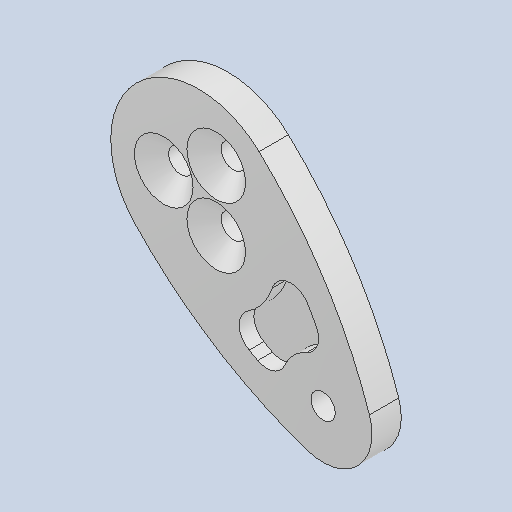
# Autodesk Inventor part: クランク_前
Saved by Autodesk Inventor 2023 (Build 270158030, 158C)
## iProperties
Created: 2022-01-08
Part Number: クランク_前
Material: Aluminum 2014-T6
Document SubType Name: Modeling
Designer: acps
Density: 2.78927 g/cm^3
Appearance: Satin
Author: acps
Autodesk Inventor part; units mm, degrees
ref_plane "YZ Plane" through (0, 0, 0) normal (1, 0, 0) x (0, 1, 0)
ref_plane "XZ Plane" through (0, 0, 0) normal (0, 1, 0) x (-1, 0, 0)
ref_plane "XY Plane" through (0, 0, 0) normal (0, 0, 1) x (1, 0, 0)
sketch "Sketch2" plane through (0, 0, 0) normal (0, 0, 1) x (1, 0, 0)
  line L0 (0, 0) -> (-12.7279, 12.7279) construction
  line L1 (0, 0) -> (18, 0) construction
  line L2 (0, 0) -> (-12.7279, 12.7279) construction
  line L3 (-3.5355, -3.5355) -> (-16.2635, 9.1924) construction
  line L4 (-9.1924, 16.2635) -> (3.5355, 3.5355) construction
  arc A0 (-3.5355, -3.5355) -> (-1.5844, -4.7423) centre (0, 0) ccw construction
  arc A1 (-9.1924, 16.2635) -> (-16.2635, 9.1924) centre (-12.7279, 12.7279) ccw
  arc A2 (-6.5476, 19.2704) -> (-19.2704, 6.5476) centre (-12.7279, 12.7279) ccw
  arc A3 (-19.2704, 6.5476) -> (-1.5844, -4.7423) centre (12.0821, 36.1644) ccw
  arc A4 (4.7423, 1.5844) -> (-6.5476, 19.2704) centre (-36.1644, -12.0821) ccw
  arc A5 (-3.9009, 10.972) -> (-6.5476, 19.2704) centre (-12.7279, 12.7279) ccw construction
  arc A6 (-6.364, 6.364) -> (-3.9009, 10.972) centre (-12.7279, 12.7279) ccw construction
  arc A7 (-10.972, 3.9009) -> (-6.364, 6.364) centre (-12.7279, 12.7279) ccw construction
  arc A8 (-19.2704, 6.5476) -> (-10.972, 3.9009) centre (-12.7279, 12.7279) ccw construction
  arc A9 (4.7423, 1.5844) -> (3.5355, 3.5355) centre (0, 0) ccw construction
  circle A10 centre (0, 0) radius 5
  circle A11 centre (0, 0) radius 3.025 construction
  circle A12 centre (0, 0) radius 1.25
  line L5 (0, 0) -> (-12.7279, 12.7279) construction
  line L6 (0, 0) -> (18, 0) construction
  line L7 (0, 0) -> (-12.7279, 12.7279) construction
  line L8 (-3.5355, -3.5355) -> (-16.2635, 9.1924) construction
  line L9 (-9.1924, 16.2635) -> (3.5355, 3.5355) construction
  arc A13 (-3.5355, -3.5355) -> (-1.5844, -4.7423) centre (0, 0) ccw construction
  arc A14 (-9.1924, 16.2635) -> (-16.2635, 9.1924) centre (-12.7279, 12.7279) ccw
  arc A15 (-6.5476, 19.2704) -> (-19.2704, 6.5476) centre (-12.7279, 12.7279) ccw
  circle A16 centre (-10.9381, 15.8279) radius 1.25
  circle A17 centre (-10.9381, 15.8279) radius 3.1 construction
  circle A18 centre (-16.3075, 12.7279) radius 1.25
  circle A19 centre (-16.3075, 12.7279) radius 3.1 construction
  circle A20 centre (-10.9381, 9.6279) radius 1.25
  circle A21 centre (-10.9381, 9.6279) radius 3.1 construction
  arc A22 (-19.2704, 6.5476) -> (-1.5844, -4.7423) centre (12.0821, 36.1644) ccw
  arc A23 (4.7423, 1.5844) -> (-6.5476, 19.2704) centre (-36.1644, -12.0821) ccw
  arc A24 (-3.9009, 10.972) -> (-6.5476, 19.2704) centre (-12.7279, 12.7279) ccw construction
  arc A25 (-6.364, 6.364) -> (-3.9009, 10.972) centre (-12.7279, 12.7279) ccw construction
  arc A26 (-10.972, 3.9009) -> (-6.364, 6.364) centre (-12.7279, 12.7279) ccw construction
  arc A27 (-19.2704, 6.5476) -> (-10.972, 3.9009) centre (-12.7279, 12.7279) ccw construction
  arc A28 (4.7423, 1.5844) -> (3.5355, 3.5355) centre (0, 0) ccw construction
  circle A29 centre (0, 0) radius 5
  circle A30 centre (0, 0) radius 3.025 construction
  circle A31 centre (0, 0) radius 1.25
  point P0 (-6.364, 6.364)
  point P1 (-11.1244, -0.1893)
  point P2 (-6.364, 6.364)
  point P3 (-11.1244, -0.1893)
  point P4 (4.7423, 1.5844)
  point P5 (-1.5844, -4.7423)
  dimension "d47" = 18
  dimension "d48" = 135
  dimension "d49" = 5
  dimension "d50" = 18
  dimension "d54" = 8
  dimension "d55" = 10
  dimension "d56" = 6.05
  dimension "d57" = 2.5
  dimension "d58" = 18
  dimension "d59" = 135
  dimension "d60" = 5
  dimension "d61" = 18
  dimension "d62" = 2.5
  dimension "d63" = 6.2
  dimension "d64" = 360
  dimension "d65" = 8
  dimension "d66" = 10
  dimension "d67" = 6.05
  dimension "d68" = 2.5
  constraints: 48 point on circle, 32 centre point, 24 end point, 17 tangent, 11 coincident, 6 equal length, 6 symmetric about line, 4 midpoint, 4 point on line, 2 horizontal, 1 vertical alignment, 17 other
  measures "d47" distance of L0.start L0.end
  measures "d48" angle of L1 L0
  measures "d49" radius of A0
  measures "d50" diameter of A2
  measures "d54" distance from line of L0 point (-11.124, -0.189)
  measures "d55" diameter of A10
  measures "d56" diameter of A11
  measures "d57" diameter of A12
  measures "d58" distance of L5.start L5.end
  measures "d59" angle of L6 L5
  measures "d60" radius of A13
  measures "d61" diameter of A15
  measures "d62" diameter of A16
  measures "d63" diameter of A17
  measures "d65" distance from line of L5 point (-11.124, -0.189)
  measures "d66" diameter of A29
  measures "d67" diameter of A30
  measures "d68" diameter of A31
extrude "Extrusion2" add sketch "Sketch2" against normal blind 3
chamfer "Chamfer3" distance 1.75 angle 45 3 edges at (-12.1881, 15.8279, 0) (-17.5575, 12.7279, 0) (-12.1881, 9.6279, 0)
sketch "Sketch3" plane through (0, 0, 0) normal (0, 0, 1) x (1, 0, 0)
  circle A0 centre (-10.9381, 9.6279) radius 3 projected
  arc A1 (-19.2704, 6.5476) -> (-1.5844, -4.7423) centre (12.0821, 36.1644) ccw projected
  circle A2 centre (0, 0) radius 1.25 projected
  arc A3 (4.7423, 1.5844) -> (-6.5476, 19.2704) centre (-36.1644, -12.0821) ccw projected
  circle A4 centre (-16.3075, 12.7279) radius 3 projected
  circle A5 centre (-10.9381, 15.8279) radius 3 projected
  arc A6 (-1.5757, 8.2644) -> (-5.2092, 7.8448) centre (-3.2996, 7.2504) ccw
  arc A7 (-7.6726, 4.5944) -> (-7.5631, 1.1727) centre (-6.584, 2.9166) ccw
  arc A8 (-7.6726, 4.5944) -> (-5.2092, 7.8448) centre (-10.9381, 9.6279) ccw
  arc A9 (-7.5631, 1.1727) -> (-6.6808, 0.6917) centre (12.0821, 36.1644) ccw
  arc A10 (-0.6917, 6.6808) -> (-1.5757, 8.2644) centre (-36.1644, -12.0821) ccw
  arc A11 (-6.6808, 0.6917) -> (-3.9071, 1.6726) centre (-5.7457, 2.4596) ccw
  arc A12 (-1.6726, 3.9071) -> (-0.6917, 6.6808) centre (-2.4596, 5.7457) ccw
  arc A13 (-1.6726, 3.9071) -> (-3.9071, 1.6726) centre (0, 0) ccw
  dimension "d77" = 3
  dimension "d78" = 2
  dimension "d79" = 2
  dimension "d80" = 3
  dimension "d81" = 3
  dimension "d82" = 2
  dimension "d83" = 2
  dimension "d84" = 3
  constraints: 16 point on circle, 8 centre point, 8 tangent, 4 concentric
  measures "d77" radial gap between concentric circles of A8 A0
  measures "d78" radius of A7
  measures "d79" radius of A6
  measures "d80" radial gap between concentric circles of A1 A9
  measures "d81" radial gap between concentric circles of A3 A10
  measures "d82" radius of A11
  measures "d83" radius of A12
  measures "d84" radial gap between concentric circles of A2 A13
extrude "Extrusion3" cut sketch "Sketch3" against normal blind 1.5 contours A10 A12 A13 A11 A9 A7 A8 A6
body "Solid2"
